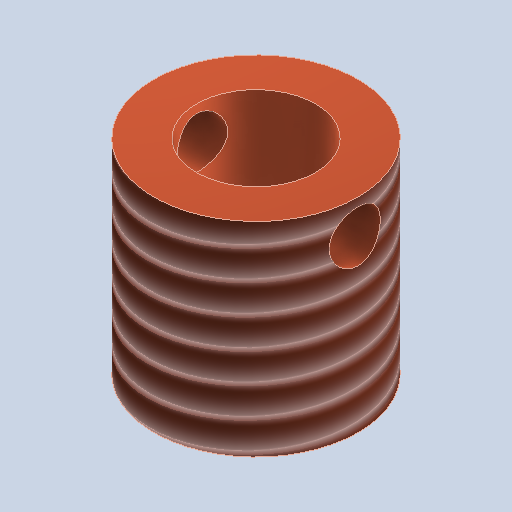
# Autodesk Inventor part: 38
Saved by Autodesk Inventor 2025.1 (Build 291241000, 241)
## iProperties
Created: 2024-09-17
Part Number: 38
Material: Copper
Document SubType Name: Modeling
Designer: ffogue
Density: 8.94 g/cm^3
Appearance: Copper - Satin
Author: ffogue
Autodesk Inventor part; units mm, degrees
ref_plane "XZ Plane" through (0, 0, 0) normal (0, 1, 0) x (-1, 0, 0)
ref_plane "XY Plane" through (0, 0, 0) normal (0, 0, 1) x (1, 0, 0)
sketch "Sketch1" plane through (0, 0, 0) normal (0, 0, 1) x (1, 0, 0)
  circle A0 centre (0, 0) radius 6
  dimension "d0" = 12
  constraints: 1 centre point, 1 coincident
  measures "d0" diameter of A0
extrude "Extrusion1" add sketch "Sketch1" along normal blind 12
thread "Thread1" size "M12x1.75" class "6g" standard "ISO Metric profile" full length
ref_plane "Work Plane1" through (6, 0, 0) normal (1, 0, 0) x (0, 1, 0)
sketch "Sketch3" plane through (6, 0, 0) normal (1, 0, 0) x (0, 1, 0)
  line L0 (6, 12) -> (-6, 12) projected
  point P0 (0, 0)
  point P1 (0, 10)
  dimension "d13" = 2
  constraints: 1 vertical alignment
  measures "d13" distance from line of L0 point (0, 10)
hole "Hole2" at (6, 0, 10) direction (-1, 0, 0) diameter 3 end through all
sketch "Sketch2" plane through (0, 0, 12) normal (0, 0, 1) x (1, 0, 0)
  circle A0 centre (0, 0) radius 6 projected
  constraints: 1 coincident
hole "Hole1" at (0, 0, 12) direction (0, 0, -1) diameter 7 depth 12
body "Solid1"
